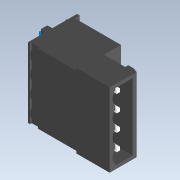
# Autodesk Inventor part: 3943133 4GD-1RR5,08-CLP-CBL
Saved by Autodesk Inventor 2021 (Build 250183000, 183)
## iProperties
Part Number: 3943133 4GD-1RR5,08-CLP-CBL
Material: Generic
Catalog Web Link: www.cadenas.de
Description: NEKM-C6 (p)-Terminal strip
Vendor: FESTO
Document SubType Name: Modeling
Designer: partserver
Manufacturer: FESTO
Mass: 4.94142 g
Surface Area: 35.2576 cm^2
Volume: 4.94142 cm^3
Density: 1 g/cm^3
Appearance: PSOLRGB-80-80-80
Categories: <MemberInstance><Categories><Category DisplayName="" Mnemonic="CABLEANDHARNESS" InternalName="e4a7e005-5e42-4d16-b293-125e7f0d0512"><Category DisplayName="" Mnemonic="CONNECTORS" InternalName="6f634eba-a678-4820-a31d-2c2d5ee6728e"><CategoryParameter DisplayName="" Mnemonic="REFDES" InternalName="c3740e8c-60ab-4d5d-8584-52b73222f2f0"/><Category DisplayName="" Mnemonic="DISCRETEWIRE" InternalName="9a3407de-09b2-4cdb-8c40-9708d5144a28"/></Category></Category></Categories><FamilyTemplate><FamilyTemplateParameters></FamilyTemplateParameters></FamilyTemplate><CategoryParameterMap><ParamToTemplateMap><ParamToTemplate CategoryParameter="//CategoryParameter[@InternalName='c3740e8c-60ab-4d5d-8584-52b73222f2f0']" ConstantValue=""/></ParamToTemplateMap></CategoryParameterMap></MemberInstance>
Category: PARTsolutions
Company: FESTO
PSOL_IDENT_0: {$CADENAS_DATA\23d-libs\festo\parts\n\nekm\parts\nekm_c6_parts.prj},199 {VTYP=3D},{NB=3943133 4GD-1R
PSOL_IDENT_1: R5,08-CLP-CBL},{LINA=3943133 4GD-1RR5,08-CLP-CBL},{NN=NEKM-C6 (p)},{DATE=16.05.2019 05:36:58},{GEOMD
PSOL_IDENT_2: ATE=16.05.2019 05:36:56},{VERSION=},{LINEID=30},{WBVAR=},{WBNUMERIC=}  {NB=3943133 4GD-1RR5,08-CLP-C
PSOL_IDENT_3: BL},{LINA=3943133 4GD-1RR5,08-CLP-CBL},{KT=DUMMY},{TNR=3943133},{TYP=4GD-1RR5,08-CLP-CBL},{VERS=2},{
PSOL_IDENT_4: N=4},{L=20.940},{L1=0.000}
NB: 3943133 4GD-1RR5,08-CLP-CBL
NN: NEKM-C6 (p)
NT: Terminal strip
NBSYN: $TNR. $TYP.
LINA: 3943133 4GD-1RR5,08-CLP-CBL
CATALOG: Festo
TNR: 3943133
TYP: 4GD-1RR5,08-CLP-CBL
VERS: 2
N: 4
L: 20.94
L1: 0
SUPPLIER: FESTO
ARTICLENO: 3943133 4GD-1RR5,08-CLP-CBL
BOMINFO: 3943133 4GD-1RR5,08-CLP-CBL
CREATOR: CADENAS GmbH
Title: 3943133 4GD-1RR5,08-CLP-CBL
Author: Cadenas PARTsolutions
Comments: Terminal strip
Autodesk Inventor part; units mm, degrees
sketch "Sketch_1" plane through (0, 0, 0) normal (0, 0, 1) x (1, 0, 0)
  line L0 (0, 6) -> (0, -7.5)
  line L1 (0, -7.5) -> (14.43, -7.5)
  arc A0 (14.43, -7.5) -> (14.73, -7.2) centre (14.43, -7.2) ccw
  line L2 (14.73, -7.2) -> (14.73, 4.1)
  arc A1 (14.73, 4.1) -> (14.73, 4.5) centre (14.73, 4.3) ccw
  line L3 (14.73, 4.5) -> (14.73, 7.2)
  arc A2 (14.73, 7.2) -> (14.43, 7.5) centre (14.43, 7.2) ccw
  line L4 (14.43, 7.5) -> (13.93, 7.5)
  line L5 (13.93, 7.5) -> (13.93, 6)
  line L6 (13.93, 6) -> (0, 6)
  constraints: 14 end point, 6 point on circle, 3 centre point
extrude "Extrusion1" add sketch "Sketch_1" along normal mid plane 20.94
sketch "Sketch_2" plane through (0, 0, 10.47) normal (0, 0, 1) x (1, 0, 0)
  line L0 (14.73, 0.2) -> (14.73, -2.756)
  arc A0 (14.9274, -2.4741) -> (14.73, -2.756) centre (15.03, -2.756) ccw
  line L1 (14.9274, -2.4741) -> (16.0326, -2.0718)
  arc A1 (16.0326, -2.0718) -> (16.23, -1.7899) centre (15.93, -1.7899) ccw
  line L2 (16.23, -1.7899) -> (16.23, -0.3)
  arc A2 (16.23, -0.3) -> (15.93, 0) centre (15.93, -0.3) ccw
  line L3 (15.93, 0) -> (14.93, 0)
  arc A3 (14.73, 0.2) -> (14.93, 0) centre (14.93, 0.2) ccw
  constraints: 8 end point, 8 point on circle, 4 centre point
extrude "Extrusion2" add sketch "Sketch_2" against normal blind 0.8
pattern_linear "Rectangular Pattern1" count 2 spacing 20.14 along (0, 0, -1) of "Extrusion2"
sketch "Sketch_4" plane through (0, 0, 5.57) normal (0, 0, 1) x (1, 0, 0)
  line L0 (14.73, 0.2) -> (14.73, -2.756)
  arc A0 (14.9274, -2.4741) -> (14.73, -2.756) centre (15.03, -2.756) ccw
  line L1 (14.9274, -2.4741) -> (16.0326, -2.0718)
  arc A1 (16.0326, -2.0718) -> (16.23, -1.7899) centre (15.93, -1.7899) ccw
  line L2 (16.23, -1.7899) -> (16.23, -0.3)
  arc A2 (16.23, -0.3) -> (15.93, 0) centre (15.93, -0.3) ccw
  line L3 (15.93, 0) -> (14.93, 0)
  arc A3 (14.73, 0.2) -> (14.93, 0) centre (14.93, 0.2) ccw
  constraints: 8 end point, 8 point on circle, 4 centre point
extrude "Extrusion3" add sketch "Sketch_4" against normal blind 0.98
pattern_linear "Rectangular Pattern2" count 3 spacing 5.08 along (0, 0, -1) of "Extrusion3"
sketch "Sketch_6" plane through (0, 0, 9.57) normal (0, 0, 1) x (1, 0, 0)
  line L0 (14.73, -2.075) -> (16.6, -2.075)
  arc A0 (16.6, -2.075) -> (16.8, -1.875) centre (16.6, -1.875) ccw
  line L1 (16.8, -1.875) -> (16.8, -1.7601)
  arc A1 (16.8, -1.7601) -> (16.6041, -1.516) centre (16.55, -1.7601) ccw
  line L2 (16.6041, -1.516) -> (15.9359, -1.3679)
  arc A2 (15.9359, -0.7821) -> (15.9359, -1.3679) centre (16.0008, -1.075) ccw
  line L3 (15.9359, -0.7821) -> (16.6041, -0.634)
  arc A3 (16.6041, -0.634) -> (16.8, -0.3899) centre (16.55, -0.3899) ccw
  line L4 (16.8, -0.3899) -> (16.8, -0.275)
  arc A4 (16.8, -0.275) -> (16.6, -0.075) centre (16.6, -0.275) ccw
  line L5 (16.6, -0.075) -> (14.73, -0.075)
  line L6 (14.73, -0.075) -> (14.73, -2.075)
  constraints: 14 end point, 10 point on circle, 5 centre point
extrude "Extrusion4" add sketch "Sketch_6" against normal blind 3.9
pattern_linear "Rectangular Pattern3" count 4 spacing 5.08 along (0, 0, -1) of "Extrusion4"
sketch "Sketch_8" plane through (0, -4.65, 0) normal (0, 1, 0) x (1, 0, 0)
  line L0 (14.73, -7.82) -> (11.73, -7.82)
  line L1 (11.73, -7.82) -> (11.73, -5.82)
  line L2 (11.73, -5.82) -> (14.53, -5.82)
  arc A0 (14.53, -5.82) -> (14.73, -5.62) centre (14.53, -5.62) ccw
  line L3 (14.73, -5.62) -> (14.73, -7.82)
  line L4 (14.73, -7.82) -> (11.73, -7.82)
  constraints: 10 end point, 2 point on circle, 1 centre point
revolve "Revolution1" cut sketch "Sketch_8" angle 360 about axis through (14.73, -4.65, 7.82) along (1, 0, 0)
pattern_linear "Rectangular Pattern4" count 4 spacing 5.08 along (0, 0, -1) of "Revolution1"
sketch "Sketch_10" plane through (13.93, 0, 0) normal (1, 0, 0) x (0, 0, -1)
  line L0 (-9.9113, 6) -> (-5.3287, 6)
  arc A0 (-5.3287, 6) -> (-9.9113, 6) centre (-7.62, 5) ccw
  constraints: 2 end point, 2 point on circle, 1 centre point
extrude "Extrusion5" add sketch "Sketch_10" against normal blind 9.7
pattern_linear "Rectangular Pattern5" count 4 spacing 5.08 along (0, 0, -1) of "Extrusion5"
sketch "Sketch_12" plane through (0, 0, 0) normal (0, 0, 1) x (1, 0, 0)
  line L0 (2, 7.5) -> (2, 6)
  line L1 (2, 6) -> (4.23, 6)
  line L2 (4.23, 6) -> (5.73, 7.5)
  line L3 (5.73, 7.5) -> (2, 7.5)
  constraints: 8 end point
extrude "Extrusion6" cut sketch "Sketch_12" along normal mid plane 20.94
sketch "Sketch_13" plane through (14.73, 0, 0) normal (1, 0, 0) x (0, 0, -1)
  line L0 (-8.795, 5.775) -> (-8.795, 4.6)
  line L1 (-8.795, 4.6) -> (-6.445, 4.6)
  line L2 (-6.445, 4.6) -> (-6.445, 5.775)
  arc A0 (-6.445, 5.775) -> (-8.795, 5.775) centre (-7.62, 5.775) ccw
  constraints: 6 end point, 2 point on circle, 1 centre point
extrude "Extrusion7" cut sketch "Sketch_13" against normal blind 9.325
pattern_linear "Rectangular Pattern6" count 4 spacing 5.08 along (0, 0, -1) of "Extrusion7"
sketch "Sketch_15" plane through (0, 7.5, 0) normal (0, 1, 0) x (1, 0, 0)
  arc A0 (5.405, -6.445) -> (5.405, -8.795) centre (5.405, -7.62) ccw
  line L0 (5.405, -8.795) -> (6.58, -8.795)
  line L1 (6.58, -8.795) -> (6.58, -6.445)
  line L2 (6.58, -6.445) -> (5.405, -6.445)
  constraints: 6 end point, 2 point on circle, 1 centre point
extrude "Extrusion8" cut sketch "Sketch_15" against normal blind 2.9
pattern_linear "Rectangular Pattern7" count 4 spacing 5.08 along (0, 0, -1) of "Extrusion8"
sketch "Sketch_17" plane through (3.13, 0, 0) normal (1, 0, 0) x (0, 0, -1)
  line L0 (-7.62, 6) -> (-7.62, 6.3)
  arc A0 (-7.17, 6) -> (-7.62, 6.3) centre (-7.6283, 5.8001) ccw
  line L1 (-7.17, 6) -> (-7.62, 6)
  line L2 (-7.62, 6) -> (-7.62, 6.3)
  constraints: 6 end point, 2 point on circle, 1 centre point
revolve "Revolution2" add sketch "Sketch_17" angle 360 about axis through (3.13, 6, 7.62) along (0, -1, 0)
pattern_linear "Rectangular Pattern8" count 4 spacing 5.08 along (0, 0, -1) of "Revolution2"
sketch "Sketch_19" plane through (0, 0, 0) normal (0, 0, 1) x (1, 0, 0)
  line L0 (-10.1, 0.5999) -> (-10.1, -7.5)
  line L1 (-10.1, -7.5) -> (0, -7.5)
  line L2 (0, -7.5) -> (0, 0.17)
  line L3 (0, 0.17) -> (-7.1, 0.17)
  line L4 (-7.1, 0.17) -> (-7.1, 1.1)
  line L5 (-7.1, 1.1) -> (-8.726, 1.1)
  line L6 (-8.726, 1.1) -> (-10.1, 0.5999)
  constraints: 14 end point
extrude "Extrusion9" add sketch "Sketch_19" along normal mid plane 22.32
sketch "Sketch_20" plane through (-1.9, 0, 0) normal (1, 0, 0) x (0, 0, -1)
  line L0 (-10.12, -5.83) -> (-9.6596, -5.83)
  arc A0 (-9.6596, -5.83) -> (-5.5804, -5.83) centre (-7.62, -3.63) ccw
  line L1 (-5.5804, -5.83) -> (-4.5796, -5.83)
  arc A1 (-4.5796, -5.83) -> (-0.5004, -5.83) centre (-2.54, -3.63) ccw
  line L2 (-0.5004, -5.83) -> (0.5004, -5.83)
  arc A2 (0.5004, -5.83) -> (4.5796, -5.83) centre (2.54, -3.63) ccw
  line L3 (4.5796, -5.83) -> (5.5804, -5.83)
  arc A3 (5.5804, -5.83) -> (9.6596, -5.83) centre (7.62, -3.63) ccw
  line L4 (9.6596, -5.83) -> (10.12, -5.83)
  line L5 (10.12, -5.83) -> (10.12, -0.537)
  line L6 (10.12, -0.537) -> (-10.12, -0.537)
  line L7 (-10.12, -0.537) -> (-10.12, -5.83)
  constraints: 16 end point, 8 point on circle, 4 centre point
extrude "Extrusion10" cut sketch "Sketch_20" against normal blind 10
sketch "Sketch_21" plane through (0, -3.63, 0) normal (0, 1, 0) x (1, 0, 0)
  line L0 (-1.9, -7.62) -> (-2.9, -7.62)
  line L1 (-2.9, -7.62) -> (-2.9, -6.22)
  line L2 (-2.9, -6.22) -> (-1.9, -6.22)
  line L3 (-1.9, -6.22) -> (-1.9, -7.62)
  line L4 (-1.9, -7.62) -> (-2.9, -7.62)
  constraints: 10 end point
revolve "Revolution3" add sketch "Sketch_21" angle 360 about axis through (-1.9, -3.63, 7.62) along (1, 0, 0)
pattern_linear "Rectangular Pattern9" count 4 spacing 5.08 along (0, 0, -1) of "Revolution3"
sketch "Sketch_23" plane through (-1.9, 0, 0) normal (1, 0, 0) x (0, 0, -1)
  line L0 (-8.12, -4.13) -> (-7.12, -4.13)
  line L1 (-7.12, -4.13) -> (-7.12, -3.13)
  line L2 (-7.12, -3.13) -> (-8.12, -3.13)
  line L3 (-8.12, -3.13) -> (-8.12, -4.13)
  constraints: 8 end point
extrude "Extrusion11" add sketch "Sketch_23" against normal blind 6.95
pattern_linear "Rectangular Pattern10" count 4 spacing 5.08 along (0, 0, -1) of "Extrusion11"
sketch "Sketch_26" plane through (-1.9, 0, 0) normal (1, 0, 0) x (0, 0, -1)
  line L0 (8.32, -2.23) -> (8.32, -5.03)
  line L1 (8.32, -5.03) -> (9.32, -5.03)
  line L2 (9.32, -5.03) -> (9.32, -2.23)
  line L3 (9.32, -2.23) -> (8.32, -2.23)
  constraints: 8 end point
extrude "Extrusion12" cut sketch "Sketch_26" against normal blind 1
sketch "Sketch_33" plane through (11.58, 0, 0) normal (1, 0, 0) x (0, 0, -1)
  line L0 (-10.47, -9) -> (10.47, -9)
  line L1 (10.47, -9) -> (10.47, -7)
  line L2 (10.47, -7) -> (9.0325, -7)
  arc A0 (5.8075, -7) -> (9.0325, -7) centre (7.42, -4.65) ccw
  line L3 (5.8075, -7) -> (3.9525, -7)
  arc A1 (0.7275, -7) -> (3.9525, -7) centre (2.34, -4.65) ccw
  line L4 (0.7275, -7) -> (-1.1275, -7)
  arc A2 (-4.3525, -7) -> (-1.1275, -7) centre (-2.74, -4.65) ccw
  line L5 (-4.3525, -7) -> (-6.2075, -7)
  arc A3 (-9.4325, -7) -> (-6.2075, -7) centre (-7.82, -4.65) ccw
  line L6 (-9.4325, -7) -> (-10.47, -7)
  line L7 (-10.47, -7) -> (-10.47, -9)
  constraints: 16 end point, 8 point on circle, 4 centre point
extrude "Extrusion13" cut sketch "Sketch_33" along normal blind 2.35
ref_plane "ANBAU_XY" through (0, 0, 0) normal (0, 1, 0) x (1, 0, 0)
ref_plane "ANBAU_YZ" through (0, 0, 0) normal (1, 0, 0) x (0, 0, -1)
ref_plane "ANBAU_ZX" through (0, 0, 0) normal (0, 0, -1) x (0, 1, 0)
ref_plane "CP1_XY" through (0, -3.63, 0) normal (1, 0, 0) x (0, 0, -1)
ref_plane "CP1_YZ" through (0, -3.63, 0) normal (0, 0, -1) x (0, 1, 0)
ref_plane "CP1_ZX" through (0, -3.63, 0) normal (0, 1, 0) x (1, 0, 0)
sketch "Sketch17" plane through (14.73, 4.1, 10.47) normal (1, 0, 0) x (0, 0, -1)
  circle A0 centre (2.65, -8.75) radius 2.2 projected
sketch "Sketch18" plane through (14.73, 4.1, 10.47) normal (1, 0, 0) x (0, 0, -1)
  circle A0 centre (7.73, -8.75) radius 2.2 projected
sketch "Sketch19" plane through (14.73, 4.1, 10.47) normal (1, 0, 0) x (0, 0, -1)
  circle A0 centre (12.81, -8.75) radius 2.2 projected
sketch "Sketch20" plane through (14.73, 4.1, 10.47) normal (1, 0, 0) x (0, 0, -1)
  circle A0 centre (17.89, -8.75) radius 2.2 projected
body "Solid1"
